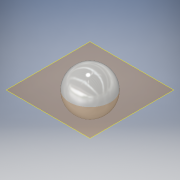
# Autodesk Inventor part: part_pinball_ece115
Saved by Autodesk Inventor 2017 (Build 210142000, 142)
## iProperties
Created: 2017-01-19
Part Number: part_pinball_ece115
Material: Generic
Document SubType Name: Modeling
Designer: John
Density: 1 g/cm^3
Appearance: Default
Author: John
Autodesk Inventor part; units mm, degrees
ref_plane "YZ Plane" through (0, 0, 0) normal (1, 0, 0) x (0, 1, 0)
ref_plane "XY Plane" through (0, 0, 0) normal (0, 0, 1) x (1, 0, 0)
sketch "Sketch1" plane through (0, 0, 0) normal (0, 1, 0) x (-1, 0, 0)
  point P0 (0, 0)
ref_plane "Work Plane1" through (0, 0, 0) normal (0, 1, 0) x (-1, 0, 0)
sketch "Sketch2" plane through (0, 0, 0) normal (0, 1, 0) x (-1, 0, 0)
  arc A0 (5.5, 0) -> (-5.5, 0) centre (0, 0) ccw construction
  line L0 (-5.5, 0) -> (5.5, 0)
  arc A1 (-5.5, 0) -> (5.5, 0) centre (0, 0) ccw
  arc A2 (-5.5, 0) -> (5.5, 0) centre (0, 0) ccw
  line L1 (7.7, 0) -> (-7.7, 0) projected
  constraints: 6 point on circle, 3 centre point, 2 coincident, 2 end point
revolve "Revolution1" add sketch "Sketch2" angle 360 about axis through (-10, 0, 0) along (1, 0, 0)
body "Solid1"
